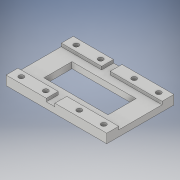
# Autodesk Inventor part: Clamps_v4_davidcell
Saved by Autodesk Inventor 2019 (Build 230136000, 136)
## iProperties
Created: 2017-09-27
Part Number: Clamps_v4_davidcell
Material: Generic
Document SubType Name: Modeling
Designer: Jonathan
Density: 1 g/cm^3
Appearance: Default
Author: Jonathan
Autodesk Inventor part; units mm, degrees
ref_plane "YZ Plane" through (0, 0, 0) normal (1, 0, 0) x (0, 1, 0)
ref_plane "XZ Plane" through (0, 0, 0) normal (0, 1, 0) x (-1, 0, 0)
ref_plane "XY Plane" through (0, 0, 0) normal (0, 0, 1) x (1, 0, 0)
sketch "Sketch1" plane through (0, 0, 0) normal (0, 1, 0) x (-1, 0, 0)
  line L0 (82.5, 55) -> (-82.5, 55)
  line L1 (-82.5, 55) -> (-82.5, -55)
  line L2 (-82.5, -55) -> (82.5, -55)
  line L3 (82.5, -55) -> (82.5, 55)
  line L4 (82.5, 55) -> (-82.5, -55) construction
  line L5 (-82.5, 55) -> (82.5, -55) construction
  point P0 (0, 0)
  dimension "d0" = 165
  dimension "d1" = 110
  constraints: 12 end point, 2 midpoint, 2 parallel, 1 horizontal, 1 perpendicular
  measures "d0" distance of L1.end L2.end
  measures "d1" distance of L2.end L0.start
extrude "Extrusion1" add sketch "Sketch1" along normal blind 15
sketch "Sketch3" plane through (0, 15, 0) normal (0, 1, 0) x (1, 0, 0)
  line L0 (82.5, -55) -> (82.5, 55) projected
  line L1 (-82.5, -35.5) -> (82.5, -35.5)
  line L2 (82.5, -35.5) -> (82.5, 35.5)
  line L3 (82.5, 35.5) -> (-82.5, 35.5)
  line L4 (-82.5, 35.5) -> (-82.5, -35.5)
  line L5 (-82.5, -35.5) -> (82.5, 35.5) construction
  line L6 (82.5, -35.5) -> (-82.5, 35.5) construction
  point P0 (0, 0)
  dimension "d8" = 71
  constraints: 12 end point, 2 midpoint, 2 parallel, 1 horizontal, 1 perpendicular, 1 point on line
  measures "d8" distance of L3.end L1.start
extrude "Extrusion3" cut sketch "Sketch3" against normal blind 5
sketch "Sketch4" plane through (0, 15, 0) normal (0, 1, 0) x (1, 0, 0)
  circle A0 centre (-67.5, -45) radius 4
  line L0 (-82.5, -55) -> (82.5, -55) projected
  line L1 (-82.5, -35.5) -> (-82.5, -55) projected
  line L2 (-82.5, -45) -> (82.5, -45)
  line L3 (82.5, -55) -> (82.5, 55) projected
  circle A1 centre (-27.5, -45) radius 4
  line L4 (-82.5, -55) -> (82.5, -55) projected
  line L5 (0, -55) -> (0, 55)
  line L6 (82.5, 55) -> (-82.5, 55) projected
  line L7 (-82.5, 55) -> (-82.5, -55) projected
  line L8 (-82.5, 0) -> (82.5, 0)
  circle A2 centre (67.5, -45) radius 4
  circle A3 centre (27.5, -45) radius 4
  circle A4 centre (-67.5, 45) radius 4
  circle A5 centre (-27.5, 45) radius 4
  circle A6 centre (67.5, 45) radius 4
  circle A7 centre (27.5, 45) radius 4
  point P0 (0, 0)
  dimension "d11" = 10
  dimension "d12" = 8
  dimension "d17" = 15
  dimension "d19" = 27.5
  constraints: 8 centre point, 6 end point, 6 symmetric about line, 4 midpoint, 4 point on line, 1 equal radius, 1 perpendicular, 6 other
  measures "d11" distance from line of L0 A0.centre
  measures "d12" diameter of A0
  measures "d17" distance from line of L1 A0.centre
  measures "d19" distance from line of L5 A1.centre
sketch "Sketch5" plane through (0, 10, 0) normal (0, 1, 0) x (1, 0, 0)
  line L0 (-52.5, -23) -> (52.5, -23)
  line L1 (52.5, -23) -> (52.5, 23)
  line L2 (52.5, 23) -> (-52.5, 23)
  line L3 (-52.5, 23) -> (-52.5, -23)
  line L4 (-52.5, -23) -> (52.5, 23) construction
  line L5 (52.5, -23) -> (-52.5, 23) construction
  line L6 (-82.5, 35.5) -> (82.5, 35.5) projected
  line L7 (-82.5, -35.5) -> (-82.5, 35.5) projected
  point P0 (0, 0)
  dimension "d13" = 12.5
  dimension "d14" = 30
  constraints: 12 end point, 2 midpoint, 2 parallel, 1 horizontal, 1 perpendicular
  measures "d13" distance between parallel lines of L6 L2
  measures "d14" distance between parallel lines of L3 L7
extrude "Extrusion4" cut sketch "Sketch5" against normal through all
extrude "Extrusion5" cut sketch "Sketch4" against normal through all contours L2 A0 | A0 L2 | A1 L2 | L2 A1 | A3 L2 | L2 A3 | A2 L2 | L2 A2 | A4 | A5 | A6 | A7
sketch "Sketch6" plane through (0, 15, 0) normal (0, 1, 0) x (1, 0, 0)
  line L0 (-82.5, -55) -> (82.5, -55) projected
  line L1 (82.5, 55) -> (-82.5, 55) projected
  line L2 (-16.5, -55) -> (-2.5, -55)
  line L3 (-2.5, -55) -> (-2.5, 55)
  line L4 (-2.5, 55) -> (-16.5, 55)
  line L5 (-16.5, 55) -> (-16.5, -55)
  line L6 (82.5, -55) -> (82.5, -35.5) projected
  point P0 (0, 0)
  dimension "d22" = 85
  dimension "d23" = 14
  constraints: 8 end point, 2 parallel, 2 point on line, 1 horizontal, 1 perpendicular
  measures "d22" distance between parallel lines of L6 L3
  measures "d23" distance between parallel lines of L3 L5
extrude "Extrusion6" cut sketch "Sketch6" against normal up to surface (5 mm away)
body "Solid1"
